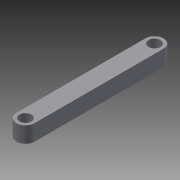
# Autodesk Inventor part: un
Saved by Autodesk Inventor 2014 SP1 (Build 180222100, 222)
## iProperties
Created: 2017-09-24
Part Number: un
Material: Generic
Document SubType Name: Modeling
Designer: Vivi
Density: 1 g/cm^3
Appearance: Default
Author: Vivi
Autodesk Inventor part; units mm, degrees
ref_plane "YZ Plane" through (0, 0, 0) normal (1, 0, 0) x (0, 1, 0)
ref_plane "XZ Plane" through (0, 0, 0) normal (0, 1, 0) x (-1, 0, 0)
ref_plane "XY Plane" through (0, 0, 0) normal (0, 0, 1) x (1, 0, 0)
sketch "Sketch1" plane through (0, 0, 0) normal (0, 0, 1) x (1, 0, 0)
  line L0 (0, 0) -> (0, 32.25) construction
  line L1 (2.25, 0) -> (2.25, 32.25)
  line L2 (-2.25, 32.25) -> (-2.25, 0)
  arc A0 (-2.25, 0) -> (2.25, 0) centre (0, 0) ccw
  arc A1 (2.25, 32.25) -> (-2.25, 32.25) centre (0, 32.25) ccw
  circle A2 centre (0, 0) radius 1.5
  circle A3 centre (0, 32.25) radius 1.5
  point P0 (0, 16.125)
  dimension "d0" = 32.25
  dimension "d1" = 4.5
  dimension "d2" = 3
  dimension "d3" = 3
  constraints: 8 end point, 4 centre point, 4 point on circle, 4 tangent, 2 coincident, 1 midpoint, 1 parallel, 1 vertical
  measures "d0" distance of L0.start L0.end
  measures "d1" diameter of A1
  measures "d2" diameter of A2
  measures "d3" diameter of A3
extrude "Extrusion1" add sketch "Sketch1" along normal mid plane 4
body "Solid1"
